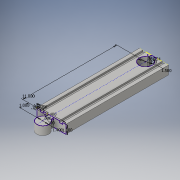
# Autodesk Inventor part: Caufield_Straight_Track
Saved by Autodesk Inventor 2016 (Build 200138000, 138)
## iProperties
Created: 2018-01-11
Part Number: Caufield_Straight_Track
Material: Generic
Document SubType Name: Modeling
Designer: caufield58738
Density: 1 g/cm^3
Appearance: Default
Author: caufield58738
Autodesk Inventor part; units mm, degrees
ref_plane "YZ Plane" through (0, 0, 0) normal (1, 0, 0) x (0, 1, 0)
ref_plane "XZ Plane" through (0, 0, 0) normal (0, 1, 0) x (-1, 0, 0)
ref_plane "XY Plane" through (0, 0, 0) normal (0, 0, 1) x (1, 0, 0)
sketch "Track sketch" plane through (0, 0, 0) normal (0, 0, 1) x (1, 0, 0)
  line L0 (0, 0) -> (86.36, 0)
  line L1 (86.36, 0) -> (86.36, 25.4)
  line L2 (0, 25.4) -> (0, 0)
  line L3 (19.05, 25.4) -> (19.05, 20.6375)
  line L4 (19.05, 20.6375) -> (10.16, 20.6375)
  line L5 (10.16, 20.6375) -> (10.16, 25.4)
  line L6 (43.18, 25.4) -> (43.18, 0) construction
  line L7 (67.31, 25.4) -> (67.31, 20.6375)
  line L8 (67.31, 20.6375) -> (76.2, 20.6375)
  line L9 (76.2, 20.6375) -> (76.2, 25.4)
  line L10 (10.16, 25.4) -> (0, 25.4)
  line L11 (86.36, 25.4) -> (76.2, 25.4)
  line L12 (67.31, 25.4) -> (19.05, 25.4)
  dimension "d0" = 86.36
  dimension "d1" = 25.4
  dimension "d2" = 19.05
  dimension "d3" = 10.16
  dimension "d6" = 4.7625
  constraints: 26 end point, 5 parallel, 4 symmetric about line, 2 collinear, 2 midpoint, 1 horizontal, 1 perpendicular
  measures "d0" distance of L2.start L1.end
  measures "d1" distance of L1.end L0.end
  measures "d2" distance between parallel lines of L3 L2
  measures "d3" distance between parallel lines of L5 L2
  measures "d6" distance of L4.end L5.end
extrude "Track extrusion" add sketch "Track sketch" against normal blind 304.8
sketch "Interlock sketch" plane through (19.05, 25.4, 0) normal (0, 1, 0) x (1, 0, 0)
  line L0 (0, 304.8) -> (48.26, 304.8) projected
  line L1 (48.26, 0) -> (0, 0) projected
  line L2 (67.31, 304.8) -> (-19.05, 304.8) construction
  line L3 (24.13, 304.8) -> (24.13, 0) construction
  arc A0 (13.693, 295.3365) -> (34.567, 295.3365) centre (24.13, 279.4) ccw
  line L4 (24.13, 0) -> (24.13, -37.5624) construction
  arc A1 (14.341, -10.5574) -> (33.919, -10.5574) centre (24.13, -25.4) ccw
  line L5 (32.385, 296.5685) -> (32.385, 296.5685)
  line L6 (15.875, 296.5685) -> (15.875, 296.5685)
  line L7 (32.385, 299.3738) -> (32.385, 304.8)
  line L8 (15.875, 299.3738) -> (15.875, 304.8)
  line L9 (15.875, 296.5685) -> (32.385, 296.5685) construction
  line L10 (16.51, 0) -> (31.75, 0)
  line L11 (31.75, 0) -> (31.75, -6.5286)
  line L12 (31.75, -9.3356) -> (16.51, -9.3356) construction
  line L13 (16.51, -6.5286) -> (16.51, 0)
  arc A2 (14.341, -10.5574) -> (16.51, -6.5286) centre (11.684, -6.5286) ccw
  arc A3 (31.75, -6.5286) -> (33.919, -10.5574) centre (36.576, -6.5286) ccw
  arc A4 (13.693, 295.3365) -> (15.875, 299.3738) centre (11.049, 299.3738) ccw
  arc A5 (32.385, 299.3738) -> (34.567, 295.3365) centre (37.211, 299.3738) ccw
  line L14 (15.875, 304.8) -> (32.385, 304.8)
  point P0 (-19.05, 0)
  dimension "d9" = 38.1
  dimension "d10" = 279.4
  dimension "d11" = 35.56
  dimension "d12" = 25.4
  dimension "d14" = 16.51
  dimension "d15" = 8.2315
  dimension "d16" = 15.24
  dimension "d17" = 4.826
  dimension "d18" = 4.826
  constraints: 24 end point, 17 point on circle, 9 point on line, 8 tangent, 6 centre point, 3 parallel, 2 equal radius, 2 horizontal, 2 midpoint, 2 perpendicular, 2 vertical, 1 collinear
  measures "d9" diameter of A0
  measures "d10" distance from line of L1 A0.centre
  measures "d11" diameter of A1
  measures "d12" distance from line of L1 A1.centre
  measures "d14" distance of L6.start L5.start
  measures "d15" distance of L5.start L7.end
  measures "d16" distance of L12.end L12.start
  measures "d17" radius of A2
  measures "d18" radius of A4
extrude "Male Interlock Extrution" add sketch "Interlock sketch" against normal blind 25.4 contours L11 A3 A1 A2 L13 L1
extrude "Female Interlock Extrusion" cut sketch "Interlock sketch" against normal blind 25.4 contours L0 L7 A5 A0 A4 L8
body "Solid1"
